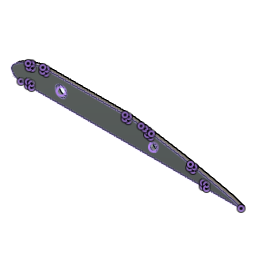
Wing rib packing tave v1.0 (Autodesk Fusion 360 design; units mm, degrees)
Autodesk Fusion 360 part; units mm, degrees
sketch "Sketch1" plane through (0, 0, 0) normal (0, 0, 1) x (1, 0, 0) in component "Airfoil structure"
  spline S0 degree 5 poles (152.8506, 9.5306) (153.6754, 9.3537) (155.1958, 9.0287) (157.0885, 8.6275) (158.936, 8.2427) (160.6637, 7.8881) (162.4454, 7.5151) (164.8303, 6.998) (168.0437, 6.2836) (171.9513, 5.3996) (176.2204, 4.4167) (180.4193, 3.4264) (184.1364, 2.5129) (187.0894, 1.7283) (189.2467, 1.0645) (190.9412, 0.4268) (192.3181, -0.1665) (193.5665, -0.7111) (194.5238, -1.126) (195.0337, -1.3464) knots 0 0 0 0 0 0 0.066667 0.133333 0.2 0.266667 0.333333 0.4 0.466667 0.533333 0.6 0.666667 0.733333 0.8 0.866667 0.933333 1 1 1 1 1 1
  line L0 (148.4907, 10.4656) -> (157.2105, 8.5955)
  line L1 (191.9852, -0.0289) -> (198.0822, -2.6639)
  circle A0 centre (33.1388, 9.1296) radius 4.765
  circle A1 centre (116.1615, 7.0362) radius 3.175
  spline S1 degree 5 poles (-3.081, -1.3464) (-3.6016, -1.2536) (-4.5414, -1.0763) (-5.6463, -0.8353) (-6.5938, -0.5669) (-7.329, -0.2953) (-8.0513, 0.0089) (-9.0194, 0.5707) (-10.0683, 1.7874) (-10.9642, 3.2518) (-11.5103, 4.4866) (-11.5777, 5.0951) (-11.407, 5.643) (-11.0112, 6.6067) (-10.1307, 7.993) (-8.6022, 9.6431) (-6.4035, 11.272) (-4.1965, 12.5715) (-2.7349, 13.4061) (-1.8316, 13.8946) (-1.0216, 14.2664) (0.0955, 14.6934) (1.459, 15.1916) (2.6392, 15.6173) (3.2971, 15.8534) knots 0 0 0 0 0 0 0.05 0.1 0.15 0.2 0.25 0.3 0.35 0.4 0.45 0.5 0.55 0.6 0.65 0.7 0.75 0.8 0.85 0.9 0.95 1 1 1 1 1 1
  line L2 (0.5703, -1.9971) -> (-6.7323, -0.6957)
  line L3 (-0.0118, 14.6656) -> (6.606, 17.0412)
  line L4 (-8.4792, 9.8153) -> (-3.9569, 12.8132)
  line L5 (-11.5034, 4.2257) -> (-11.5345, 5.6935)
  line L6 (-7.2174, -0.5359) -> (-9.7443, 1.1286)
  line L7 (19.5688, 19.3646) -> (90.5688, 19.3646)
  spline S2 degree 5 poles (93.5688, 19.3646) (93.8188, 19.3387) (94.2829, 19.2905) (94.8714, 19.229) (95.4658, 19.1659) (96.0263, 19.1049) (96.567, 19.0445) (97.2368, 18.9678) (98.1315, 18.8622) (99.313, 18.7173) (100.8214, 18.5245) (102.3118, 18.3263) (103.5973, 18.1504) (104.53, 18.0207) (105.0153, 17.9528) knots 0 0 0 0 0 0 0.1 0.2 0.3 0.4 0.5 0.6 0.7 0.8 0.9 1 1 1 1 1 1
  line L8 (92.266, 19.4996) -> (94.8715, 19.2297)
  line L9 (103.6448, 18.1447) -> (106.3858, 17.761)
  spline S3 degree 5 poles (6.5765, 16.943) (6.9079, 17.0449) (7.5374, 17.2364) (8.3817, 17.4868) (9.3156, 17.7508) (10.2084, 17.9865) (10.8922, 18.156) (11.4504, 18.29) (11.9864, 18.4184) (12.6265, 18.5675) (13.504, 18.76) (14.4962, 18.9637) (15.447, 19.1503) (16.1786, 19.2906) (16.5688, 19.3646) knots 0 0 0 0 0 0 0.1 0.2 0.3 0.4 0.5 0.6 0.7 0.8 0.9 1 1 1 1 1 1
  line L10 (5.4107, 16.5846) -> (7.7424, 17.3015)
  line L11 (15.2328, 19.111) -> (17.9048, 19.6183)
  line L12 (152.4045, 9.626) -> (152.8506, 9.5306)
  line L13 (107.9851, 17.5282) -> (108.4359, 17.4637)
  line L14 (6.1441, 16.7993) -> (6.5765, 16.943)
  line L15 (128.8588, -1.3464) -> (132.3138, -1.3464)
  line L16 (149.471, 10.2539) -> (148.8431, 7.3203)
  line L17 (148.8431, 7.3203) -> (151.7767, 6.6925)
  line L18 (151.7767, 6.6925) -> (152.4045, 9.626)
  line L19 (3.2971, 15.8534) -> (4.243, 13.0064)
  line L20 (4.243, 13.0064) -> (7.09, 13.9524)
  line L21 (7.09, 13.9524) -> (6.1441, 16.7993)
  line L22 (160.8934, -1.3464) -> (160.8934, 1.6536)
  line L23 (160.8934, 1.6536) -> (163.8934, 1.6536)
  line L24 (163.8934, 1.6536) -> (163.8934, -1.3464)
  line L25 (132.3138, -1.3464) -> (160.8934, -1.3464)
  line L26 (163.8934, -1.3464) -> (195.0337, -1.3464)
  line L27 (3.4513, -1.3464) -> (3.4513, 1.6536)
  line L28 (3.4513, 1.6536) -> (6.4513, 1.6536)
  line L29 (6.4513, 1.6536) -> (6.4513, -1.3464)
  line L30 (-3.081, -1.3464) -> (3.4513, -1.3464)
  line L31 (6.4513, -1.3464) -> (128.8588, -1.3464)
  line L32 (105.0153, 17.9528) -> (107.9851, 17.5282)
  line L33 (19.5688, 19.3646) -> (19.5688, 16.3646)
  line L34 (19.5688, 16.3646) -> (16.5688, 16.3646)
  line L35 (16.5688, 16.3646) -> (16.5688, 19.3646)
  line L36 (90.5688, 19.3646) -> (90.5688, 16.3646)
  line L37 (90.5688, 16.3646) -> (93.5688, 16.3646)
  line L38 (93.5688, 16.3646) -> (93.5688, 19.3646)
  line L39 (113.7881, 13.5683) -> (110.8279, 14.0557)
  line L40 (110.8279, 14.0557) -> (111.3153, 17.0159)
  line L41 (113.7881, 13.5683) -> (114.2755, 16.5285)
  spline S4 degree 5 poles (108.4359, 17.4637) (108.6467, 17.433) (108.9931, 17.3831) (109.2865, 17.3426) (109.4547, 17.3194) (110.0313, 17.2264) (110.7239, 17.113) (111.2088, 17.0334) (111.3153, 17.0159) knots 0 0 0 0 0 0 0.066667 0.133333 0.2 0.217791 0.217791 0.217791 0.217791 0.217791 0.217791
  line L42 (107.9387, 17.5361) -> (108.933, 17.3913)
  line L43 (110.8712, 17.0888) -> (111.7595, 16.9429)
  spline S5 degree 5 poles (114.2755, 16.5285) (114.6969, 16.4591) (115.8472, 16.2695) (117.9388, 15.9249) (121.2621, 15.3773) (125.9027, 14.6124) (130.8234, 13.7994) (135.1309, 13.0827) (138.47, 12.5166) (140.7881, 12.1042) (142.4392, 11.78) (143.9897, 11.4433) (145.6466, 11.0766) (147.3521, 10.7068) (148.7253, 10.4127) (149.471, 10.2539) knots 0.291405 0.291405 0.291405 0.291405 0.291405 0.291405 0.333333 0.4 0.466667 0.533333 0.6 0.666667 0.733333 0.8 0.866667 0.933333 1 1 1 1 1 1
  line L44 (111.4536, 16.9935) -> (117.0973, 16.0636)
  line L45 (143.5745, 11.5101) -> (155.3674, 8.9976)
  point P0 (-8.4808, 0.2964)
  point P1 (-11.5189, 4.9596)
  point P2 (-6.2181, 11.3142)
  point P3 (11.4183, 18.2822)
  point P4 (96.5722, 19.0435)
  point P5 (109.7229, 17.2753)
  point P6 (137.8507, 12.6179)
  point P7 (163.7248, 7.2358)
  point P8 (186.791, 1.7868)
  dimension "d38" = 77
  dimension "d53" = 9.53
  dimension "d54" = 6.35
  dimension "d59" = 3
  constraint midpoint S0.start L0
  constraint midpoint S0.end L1
  constraint midpoint S1.start L2
  constraint midpoint S1.end L3
  constraint midpoint P2 L4
  constraint midpoint P1 L5
  constraint midpoint P0 L6
  constraint horizontal L7
  constraint midpoint S2.start L8
  constraint midpoint S2.end L9
  constraint midpoint S3.start L10
  constraint midpoint S3.end L11
  constraint parallel L25 L30
  constraint collinear L25 L30
  constraint horizontal L30
  constraint parallel L15 L25
  constraint perpendicular L12 L16
  constraint perpendicular L16 L17
  constraint perpendicular L12 L18
  constraint perpendicular L14 L19
  constraint perpendicular L19 L20
  constraint perpendicular L14 L21
  constraint perpendicular L22 L25
  constraint perpendicular L22 L23
  constraint perpendicular L23 L24
  constraint collinear L25 L26
  constraint perpendicular L27 L30
  constraint perpendicular L27 L28
  constraint coincident L29.end L30
  constraint perpendicular L29 L30
  constraint collinear L30 L31
  constraint vertical L33
  constraint horizontal L34
  constraint vertical L35
  constraint vertical L36
  constraint horizontal L37
  constraint vertical L38
  constraint equal L36 L38
  constraint equal L36 L37
  constraint perpendicular L39 L40
  constraint perpendicular L39 L41
  constraint midpoint L13.end L42
  constraint midpoint L40.end L43
  constraint midpoint L41.end L44
  constraint midpoint L16.start L45
  measures "d38" distance of S3.end S2.start
  measures "d53" diameter of A0
  measures "d54" diameter of A1
  measures "d59" distance of L36.end L37.end
extrude "Extrude2" add sketch "Sketch1" along normal blind 3 contours S0 L0 L1 S1 L7 S2 L8 L9 S3 L12 L13 L14 L15 L16 L17 L18 L19 L20 L21 L22 L23 L24 L25 L26 L27 L28 L29 L30 L31 L32 L33 L34 L35 L36 L37 L38 L39 L40 L41 S4 L42 L43 S5 L44
sketch "lazercut" plane through (0, 0, 3) normal (0, 0, 1) x (1, 0, 0)
  circle A0 centre (33.1388, 9.1296) radius 4.765
  circle A1 centre (116.1615, 7.0362) radius 3.175
  line L0 (113.7881, 13.5683) -> (110.8279, 14.0557)
  line L1 (110.8279, 14.0557) -> (111.3153, 17.0159)
  spline S0 degree 5 poles (111.3153, 17.0159) (111.2088, 17.0334) (110.7239, 17.113) (110.0313, 17.2264) (109.4547, 17.3194) (109.2865, 17.3426) (108.9931, 17.3831) (108.6467, 17.433) (108.4359, 17.4637) knots -0.217791 -0.217791 -0.217791 -0.217791 -0.217791 -0.217791 -0.2 -0.133333 -0.066667 0 0 0 0 0 0
  line L2 (108.4359, 17.4637) -> (105.0153, 17.9528)
  spline S1 degree 5 poles (105.0153, 17.9528) (104.53, 18.0207) (103.5973, 18.1504) (102.3118, 18.3263) (100.8214, 18.5245) (99.313, 18.7173) (98.1315, 18.8622) (97.2368, 18.9678) (96.567, 19.0445) (96.0263, 19.1049) (95.4658, 19.1659) (94.8714, 19.229) (94.2829, 19.2905) (93.8188, 19.3387) (93.5688, 19.3646) knots -1 -1 -1 -1 -1 -1 -0.9 -0.8 -0.7 -0.6 -0.5 -0.4 -0.3 -0.2 -0.1 0 0 0 0 0 0
  line L3 (93.5688, 19.3646) -> (93.5688, 16.3646)
  line L4 (93.5688, 16.3646) -> (90.5688, 16.3646)
  line L5 (90.5688, 16.3646) -> (90.5688, 19.3646)
  line L6 (90.5688, 19.3646) -> (19.5688, 19.3646)
  line L7 (19.5688, 19.3646) -> (19.5688, 16.3646)
  line L8 (19.5688, 16.3646) -> (16.5688, 16.3646)
  line L9 (16.5688, 16.3646) -> (16.5688, 19.3646)
  spline S2 degree 5 poles (16.5688, 19.3646) (16.1786, 19.2906) (15.447, 19.1503) (14.4962, 18.9637) (13.504, 18.76) (12.6265, 18.5675) (11.9864, 18.4184) (11.4504, 18.29) (10.8922, 18.156) (10.2084, 17.9865) (9.3156, 17.7508) (8.3817, 17.4868) (7.5374, 17.2364) (6.9079, 17.0449) (6.5765, 16.943) knots -1 -1 -1 -1 -1 -1 -0.9 -0.8 -0.7 -0.6 -0.5 -0.4 -0.3 -0.2 -0.1 0 0 0 0 0 0
  line L10 (6.5765, 16.943) -> (6.1441, 16.7993)
  line L11 (6.1441, 16.7993) -> (7.09, 13.9524)
  line L12 (7.09, 13.9524) -> (4.243, 13.0064)
  line L13 (4.243, 13.0064) -> (3.2971, 15.8534)
  spline S3 degree 5 poles (3.2971, 15.8534) (2.6392, 15.6173) (1.459, 15.1916) (0.0955, 14.6934) (-1.0216, 14.2664) (-1.8316, 13.8946) (-2.7349, 13.4061) (-4.1965, 12.5715) (-6.4035, 11.272) (-8.6022, 9.6431) (-10.1307, 7.993) (-11.0112, 6.6067) (-11.407, 5.643) (-11.5777, 5.0951) (-11.5103, 4.4866) (-10.9642, 3.2518) (-10.0683, 1.7874) (-9.0194, 0.5707) (-8.0513, 0.0089) (-7.329, -0.2953) (-6.5938, -0.5669) (-5.6463, -0.8353) (-4.5414, -1.0763) (-3.6016, -1.2536) (-3.081, -1.3464) knots -1 -1 -1 -1 -1 -1 -0.95 -0.9 -0.85 -0.8 -0.75 -0.7 -0.65 -0.6 -0.55 -0.5 -0.45 -0.4 -0.35 -0.3 -0.25 -0.2 -0.15 -0.1 -0.05 0 0 0 0 0 0
  line L14 (-3.081, -1.3464) -> (3.4513, -1.3464)
  line L15 (3.4513, -1.3464) -> (3.4513, 1.6536)
  line L16 (3.4513, 1.6536) -> (6.4513, 1.6536)
  line L17 (6.4513, 1.6536) -> (6.4513, -1.3464)
  line L18 (6.4513, -1.3464) -> (160.8934, -1.3464)
  line L19 (160.8934, -1.3464) -> (160.8934, 1.6536)
  line L20 (160.8934, 1.6536) -> (163.8934, 1.6536)
  line L21 (163.8934, 1.6536) -> (163.8934, -1.3464)
  line L22 (163.8934, -1.3464) -> (195.0337, -1.3464)
  spline S4 degree 5 poles (195.0337, -1.3464) (194.5238, -1.126) (193.5665, -0.7111) (192.3181, -0.1665) (190.9412, 0.4268) (189.2467, 1.0645) (187.0894, 1.7283) (184.1364, 2.5129) (180.4193, 3.4264) (176.2204, 4.4167) (171.9513, 5.3996) (168.0437, 6.2836) (164.8303, 6.998) (162.4454, 7.5151) (160.6637, 7.8881) (158.936, 8.2427) (157.0885, 8.6275) (155.1958, 9.0287) (153.6754, 9.3537) (152.8506, 9.5306) knots -1 -1 -1 -1 -1 -1 -0.933333 -0.866667 -0.8 -0.733333 -0.666667 -0.6 -0.533333 -0.466667 -0.4 -0.333333 -0.266667 -0.2 -0.133333 -0.066667 0 0 0 0 0 0
  line L23 (152.8506, 9.5306) -> (152.4045, 9.626)
  line L24 (152.4045, 9.626) -> (151.7767, 6.6925)
  line L25 (151.7767, 6.6925) -> (148.8431, 7.3203)
  line L26 (148.8431, 7.3203) -> (149.471, 10.2539)
  spline S5 degree 5 poles (149.471, 10.2539) (148.7253, 10.4127) (147.3521, 10.7068) (145.6466, 11.0766) (143.9897, 11.4433) (142.4392, 11.78) (140.7881, 12.1042) (138.47, 12.5166) (135.1309, 13.0827) (130.8234, 13.7994) (125.9027, 14.6124) (121.2621, 15.3773) (117.9388, 15.9249) (115.8472, 16.2695) (114.6969, 16.4591) (114.2755, 16.5285) knots -1 -1 -1 -1 -1 -1 -0.933333 -0.866667 -0.8 -0.733333 -0.666667 -0.6 -0.533333 -0.466667 -0.4 -0.333333 -0.291405 -0.291405 -0.291405 -0.291405 -0.291405 -0.291405
  line L27 (114.2755, 16.5285) -> (113.7881, 13.5683)
sketch "Sketch3" plane through (0, 0, 0) normal (0, 0, 1) x (1, 0, 0)
component "Airfoil structure" placed x (1, 0, 0) y (0, 1, 0) z (0, 0, 1) at (0, 0, 0)
